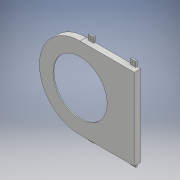
# Autodesk Inventor part: Socle
Saved by Autodesk Inventor 2018 (Build 220112000, 112)
## iProperties
Created: 2018-03-19
Part Number: Socle
Material: Générique
Document SubType Name: Modeling
Designer: Youri
Density: 1 g/cm^3
Appearance: Par défaut
Author: Youri
Autodesk Inventor part; units mm, degrees
ref_plane "YZ Plane" through (0, 0, 0) normal (1, 0, 0) x (0, 1, 0)
ref_plane "XZ Plane" through (0, 0, 0) normal (0, 1, 0) x (-1, 0, 0)
ref_plane "XY Plane" through (0, 0, 0) normal (0, 0, 1) x (1, 0, 0)
sketch "Esquisse1" plane through (0, 0, 0) normal (0, 1, 0) x (-1, 0, 0)
  line L0 (0, 0) -> (120, 0)
  line L1 (120, 180) -> (0, 180)
  line L2 (0, 180) -> (0, 0)
  arc A0 (120, 0) -> (120, 180) centre (120, 90) ccw
  circle A1 centre (120, 90) radius 60
  line L3 (120, 177) -> (3, 177)
  line L4 (3, 177) -> (3, 3)
  line L5 (3, 3) -> (120, 3)
  arc A2 (120, 3) -> (120, 177) centre (120, 90) ccw
  dimension "d2" = 120
  dimension "d3" = 120
  dimension "d4" = 180
  dimension "d5" = 3
  constraints: 12 end point, 4 point on circle, 3 centre point, 2 parallel, 1 coincident, 1 horizontal, 3 other
  measures "d2" distance of L1.start L1.end
  measures "d3" diameter of A1
  measures "d4" distance of L1.end L0.start
  measures "d5" radial gap between concentric circles of A0 A2
extrude "Extrusion1" add sketch "Esquisse1" along normal blind 2 contours L2 L1 A0 L0 | A2 L5 L4 L3
sketch "Esquisse2" plane through (0, 2, 0) normal (0, 1, 0) x (1, 0, 0)
  arc A0 (-120, 0) -> (-120, -180) centre (-120, -90) ccw projected
  arc A1 (-120, 0) -> (-120, -180) centre (-120, -90) ccw
  line L0 (-120, -180) -> (0, -180) projected
  line L1 (-120, -180) -> (0, -180)
  line L2 (0, -180) -> (0, 0)
  line L3 (0, 0) -> (-120, 0) projected
  line L4 (0, 0) -> (-120, 0)
  arc A2 (-120, -3) -> (-120, -177) centre (-120, -90) ccw
  line L5 (-120, -3) -> (0, -3)
  line L6 (-3, -3) -> (-3, -177)
  line L7 (-3, -177) -> (-120, -177)
  arc A3 (-120, -3) -> (-120, -177) centre (-120, -90) ccw
  line L8 (-120, -3) -> (-3, -3)
  dimension "d8" = 3
  dimension "d9" = 90
  dimension "d10" = 3
  constraints: 14 end point, 6 point on circle, 4 perpendicular, 3 centre point, 1 horizontal, 4 other
  measures "d8" radial gap between concentric circles of A0 A2
  measures "d9" radius of A0
  measures "d10" distance between parallel lines of L2 L6
extrude "Extrusion2" add sketch "Esquisse2" along normal blind 12
sketch "Esquisse3" plane through (0, 14, 0) normal (0, 1, 0) x (1, 0, 0)
  line L0 (-120, -180) -> (0, -180) projected
  line L1 (-7.3436, -180) -> (-19.3436, -180)
  line L2 (-19.3436, -180) -> (-19.3436, -192)
  line L3 (-19.3436, -192) -> (-7.3436, -192)
  line L4 (-7.3436, -192) -> (-7.3436, -180)
  circle A0 centre (-13.3436, -186) radius 2
  circle A1 centre (-120, -90) radius 60 projected
  line L5 (-120, -90) -> (-228.3107, -90)
  line L6 (-19.3436, 0) -> (-19.3436, 12)
  line L7 (-19.3436, 12) -> (-7.3436, 12)
  line L8 (-7.3436, 12) -> (-7.3436, 0)
  circle A2 centre (-13.3436, 6) radius 2
  line L9 (-60, -180) -> (-60, 26.6941)
  line L10 (-112.6564, -180) -> (-100.6564, -180)
  line L11 (-100.6564, -180) -> (-100.6564, -192)
  line L12 (-100.6564, -192) -> (-112.6564, -192)
  line L13 (-112.6564, -192) -> (-112.6564, -180)
  circle A3 centre (-106.6564, -186) radius 2
  line L14 (-100.6564, 12) -> (-112.6564, 12)
  line L15 (-112.6564, 12) -> (-112.6564, 0)
  circle A4 centre (-106.6564, 6) radius 2
  line L16 (-100.6564, 12) -> (-100.6564, 0)
  line L17 (0, 0) -> (-120, 0) projected
  line L18 (-7.3436, 0) -> (-19.3436, 0)
  dimension "d13" = 12
  dimension "d14" = 12
  dimension "d15" = 4
  constraints: 34 end point, 14 symmetric about line, 4 centre point, 2 horizontal, 2 parallel, 2 point on line, 2 vertical, 1 collinear, 1 midpoint, 1 perpendicular, 3 other
  measures "d13" distance of L1.end L2.end
  measures "d14" distance of L2.end L3.end
  measures "d15" diameter of A0
extrude "Extrusion3" add sketch "Esquisse3" against normal blind 3 contours L17 L15 L14 L16 | L6 L7 L8 L17 | L0 L4 L3 L2 | L0 L11 L12 L13
